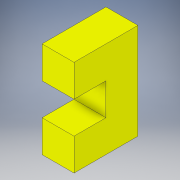
# Autodesk Inventor part: Yellow part
Saved by Autodesk Inventor 2017 (Build 210142000, 142)
## iProperties
Created: 2016-11-01
Part Number: Yellow part
Material: Generic
Document SubType Name: Modeling
Designer: rbibb
Density: 1 g/cm^3
Appearance: Default
Author: rbibb
Autodesk Inventor part; units mm, degrees
ref_plane "YZ Plane" through (0, 0, 0) normal (1, 0, 0) x (0, 1, 0)
ref_plane "XZ Plane" through (0, 0, 0) normal (0, 1, 0) x (-1, 0, 0)
ref_plane "XY Plane" through (0, 0, 0) normal (0, 0, 1) x (1, 0, 0)
sketch "Sketch1" plane through (0, 0, 0) normal (1, 0, 0) x (0, 1, 0)
  line L0 (15.1684, 31.959) -> (-41.9816, 31.959)
  line L1 (-41.9816, 31.959) -> (-41.9816, 12.909)
  line L2 (-41.9816, 12.909) -> (15.1684, 12.909)
  line L3 (15.1684, 12.909) -> (15.1684, 31.959)
  point P0 (0, 0)
  dimension "d0" = 57.15
  dimension "d1" = 19.05
  constraints: 8 end point, 2 parallel, 1 horizontal, 1 perpendicular
  measures "d0" distance of L2.end L1.end
  measures "d1" distance of L1.end L0.end
extrude "Extrusion1" add sketch "Sketch1" along normal blind 19.05
sketch "Sketch2" plane through (0, -41.9816, 31.959) normal (0, 0, 1) x (1, 0, 0)
  line L0 (0, 57.15) -> (0, 0) projected
  line L1 (19.05, 57.15) -> (19.05, 0) projected
  line L2 (0, 57.15) -> (19.05, 57.15)
  line L3 (19.05, 57.15) -> (19.05, 38.1)
  line L4 (19.05, 38.1) -> (0, 38.1)
  line L5 (0, 38.1) -> (0, 57.15)
  line L6 (0, 0) -> (19.05, 0) projected
  line L7 (0, 0) -> (19.05, 0)
  line L8 (19.05, 0) -> (19.05, 19.05)
  line L9 (19.05, 19.05) -> (0, 19.05)
  line L10 (0, 19.05) -> (0, 0)
  point P0 (0, 41.9816)
  dimension "d4" = 19.05
  dimension "d5" = 19.05
  dimension "d6" = 19.05
  constraints: 16 end point, 4 parallel, 2 horizontal, 2 perpendicular, 1 point on line
  measures "d4" distance of L2.end L3.end
  measures "d5" distance of L9.end L8.end
  measures "d6" distance of L8.end L7.end
extrude "Extrusion2" add sketch "Sketch2" along normal blind 19.05 contours L2 L1 L4 L0 | L9 L1 L6 L0
body "Solid1"
